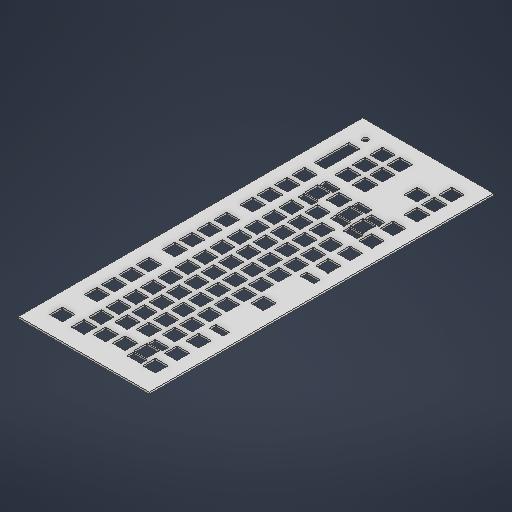
# Autodesk Inventor part: Keyboard-top
Saved by Autodesk Inventor 2026.1 (Build 301233000, 233)
## iProperties
Created: 2025-12-15
Part Number: Keyboard-top
Material: Generic
Document SubType Name: Modeling
Designer: chest
Density: 1 g/cm^3
Appearance: Default
Author: chest
Autodesk Inventor part; units mm, degrees
(part 1 of 5)
ref_plane "YZ Plane" through (0, 0, 0) normal (1, 0, 0) x (0, 1, 0)
ref_plane "XZ Plane" through (0, 0, 0) normal (0, 1, 0) x (-1, 0, 0)
ref_plane "XY Plane" through (0, 0, 0) normal (0, 0, 1) x (1, 0, 0)
sketch "Block1" plane through (0, 0, 0) normal (0, 0, 1) x (1, 0, 0)
  line L0 (31.1, 3.025) -> (31.1, 16.025)
  line L1 (45.1, 3.025) -> (45.1, 16.025)
  line L2 (31.6, 2.525) -> (44.6, 2.525)
  line L3 (31.6, 16.525) -> (44.6, 16.525)
  arc A0 (31.1, 3.025) -> (31.6, 2.525) centre (31.6, 3.025) ccw
  arc A1 (31.6, 16.525) -> (31.1, 16.025) centre (31.6, 16.025) ccw
  arc A2 (44.6, 2.525) -> (45.1, 3.025) centre (44.6, 3.025) ccw
  arc A3 (45.1, 16.025) -> (44.6, 16.525) centre (44.6, 16.025) ccw
  line L4 (31.1, 22.075) -> (31.1, 35.075)
  line L5 (45.1, 22.075) -> (45.1, 35.075)
  line L6 (31.6, 21.575) -> (44.6, 21.575)
  line L7 (31.6, 35.575) -> (44.6, 35.575)
  arc A4 (31.1, 22.075) -> (31.6, 21.575) centre (31.6, 22.075) ccw
  arc A5 (31.6, 35.575) -> (31.1, 35.075) centre (31.6, 35.075) ccw
  arc A6 (44.6, 21.575) -> (45.1, 22.075) centre (44.6, 22.075) ccw
  arc A7 (45.1, 35.075) -> (44.6, 35.575) centre (44.6, 35.075) ccw
  line L8 (31.1, 41.125) -> (31.1, 54.125)
  line L9 (45.1, 41.125) -> (45.1, 54.125)
  line L10 (31.6, 40.625) -> (44.6, 40.625)
  line L11 (31.6, 54.625) -> (44.6, 54.625)
  arc A8 (31.1, 41.125) -> (31.6, 40.625) centre (31.6, 41.125) ccw
  arc A9 (31.6, 54.625) -> (31.1, 54.125) centre (31.6, 54.125) ccw
  arc A10 (44.6, 40.625) -> (45.1, 41.125) centre (44.6, 41.125) ccw
  arc A11 (45.1, 54.125) -> (44.6, 54.625) centre (44.6, 54.125) ccw
  line L12 (31.1, 60.175) -> (31.1, 73.175)
  line L13 (45.1, 60.175) -> (45.1, 73.175)
  line L14 (31.6, 59.675) -> (44.6, 59.675)
  line L15 (31.6, 73.675) -> (44.6, 73.675)
  arc A12 (31.1, 60.175) -> (31.6, 59.675) centre (31.6, 60.175) ccw
  arc A13 (31.6, 73.675) -> (31.1, 73.175) centre (31.6, 73.175) ccw
  arc A14 (44.6, 59.675) -> (45.1, 60.175) centre (44.6, 60.175) ccw
  arc A15 (45.1, 73.175) -> (44.6, 73.675) centre (44.6, 73.175) ccw
  line L16 (31.1, 79.225) -> (31.1, 92.225)
  line L17 (45.1, 79.225) -> (45.1, 92.225)
  line L18 (31.6, 78.725) -> (44.6, 78.725)
  line L19 (31.6, 92.725) -> (44.6, 92.725)
  arc A16 (31.1, 79.225) -> (31.6, 78.725) centre (31.6, 79.225) ccw
  arc A17 (31.6, 92.725) -> (31.1, 92.225) centre (31.6, 92.225) ccw
  arc A18 (44.6, 78.725) -> (45.1, 79.225) centre (44.6, 79.225) ccw
  arc A19 (45.1, 92.225) -> (44.6, 92.725) centre (44.6, 92.225) ccw
  line L20 (31.1, 98.275) -> (31.1, 111.275)
  line L21 (45.1, 98.275) -> (45.1, 111.275)
  line L22 (31.6, 97.775) -> (44.6, 97.775)
  line L23 (31.6, 111.775) -> (44.6, 111.775)
  arc A20 (31.1, 98.275) -> (31.6, 97.775) centre (31.6, 98.275) ccw
  arc A21 (31.6, 111.775) -> (31.1, 111.275) centre (31.6, 111.275) ccw
  arc A22 (44.6, 97.775) -> (45.1, 98.275) centre (44.6, 98.275) ccw
  arc A23 (45.1, 111.275) -> (44.6, 111.775) centre (44.6, 111.275) ccw
  line L24 (31.1, 117.325) -> (31.1, 130.325)
  line L25 (45.1, 117.325) -> (45.1, 130.325)
  line L26 (31.6, 116.825) -> (44.6, 116.825)
  line L27 (31.6, 130.825) -> (44.6, 130.825)
  arc A24 (31.1, 117.325) -> (31.6, 116.825) centre (31.6, 117.325) ccw
  arc A25 (31.6, 130.825) -> (31.1, 130.325) centre (31.6, 130.325) ccw
  arc A26 (44.6, 116.825) -> (45.1, 117.325) centre (44.6, 117.325) ccw
  arc A27 (45.1, 130.325) -> (44.6, 130.825) centre (44.6, 130.325) ccw
  line L28 (31.1, 136.375) -> (31.1, 149.375)
  line L29 (45.1, 136.375) -> (45.1, 149.375)
  line L30 (31.6, 135.875) -> (44.6, 135.875)
  line L31 (31.6, 149.875) -> (44.6, 149.875)
  arc A28 (31.1, 136.375) -> (31.6, 135.875) centre (31.6, 136.375) ccw
  arc A29 (31.6, 149.875) -> (31.1, 149.375) centre (31.6, 149.375) ccw
  arc A30 (44.6, 135.875) -> (45.1, 136.375) centre (44.6, 136.375) ccw
  arc A31 (45.1, 149.375) -> (44.6, 149.875) centre (44.6, 149.375) ccw
  line L32 (31.1, 155.425) -> (31.1, 168.425)
  line L33 (45.1, 155.425) -> (45.1, 168.425)
  line L34 (31.6, 154.925) -> (44.6, 154.925)
  line L35 (31.6, 168.925) -> (44.6, 168.925)
  arc A32 (31.1, 155.425) -> (31.6, 154.925) centre (31.6, 155.425) ccw
  arc A33 (31.6, 168.925) -> (31.1, 168.425) centre (31.6, 168.425) ccw
  arc A34 (44.6, 154.925) -> (45.1, 155.425) centre (44.6, 155.425) ccw
  arc A35 (45.1, 168.425) -> (44.6, 168.925) centre (44.6, 168.425) ccw
  line L36 (31.1, 174.475) -> (31.1, 187.475)
  line L37 (45.1, 174.475) -> (45.1, 187.475)
  line L38 (31.6, 173.975) -> (44.6, 173.975)
  line L39 (31.6, 187.975) -> (44.6, 187.975)
  arc A36 (31.1, 174.475) -> (31.6, 173.975) centre (31.6, 174.475) ccw
  arc A37 (31.6, 187.975) -> (31.1, 187.475) centre (31.6, 187.475) ccw
  arc A38 (44.6, 173.975) -> (45.1, 174.475) centre (44.6, 174.475) ccw
  arc A39 (45.1, 187.475) -> (44.6, 187.975) centre (44.6, 187.475) ccw
  line L40 (31.1, 193.525) -> (31.1, 206.525)
  line L41 (45.1, 193.525) -> (45.1, 206.525)
  line L42 (31.6, 193.025) -> (44.6, 193.025)
  line L43 (31.6, 207.025) -> (44.6, 207.025)
  arc A40 (31.1, 193.525) -> (31.6, 193.025) centre (31.6, 193.525) ccw
  arc A41 (31.6, 207.025) -> (31.1, 206.525) centre (31.6, 206.525) ccw
  arc A42 (44.6, 193.025) -> (45.1, 193.525) centre (44.6, 193.525) ccw
  arc A43 (45.1, 206.525) -> (44.6, 207.025) centre (44.6, 206.525) ccw
  line L44 (31.1, 212.575) -> (31.1, 225.575)
  line L45 (45.1, 212.575) -> (45.1, 225.575)
  line L46 (31.6, 212.075) -> (44.6, 212.075)
  line L47 (31.6, 226.075) -> (44.6, 226.075)
  arc A44 (31.1, 212.575) -> (31.6, 212.075) centre (31.6, 212.575) ccw
  arc A45 (31.6, 226.075) -> (31.1, 225.575) centre (31.6, 225.575) ccw
  arc A46 (44.6, 212.075) -> (45.1, 212.575) centre (44.6, 212.575) ccw
  arc A47 (45.1, 225.575) -> (44.6, 226.075) centre (44.6, 225.575) ccw
  line L48 (31.1, 231.625) -> (31.1, 244.625)
  line L49 (45.1, 231.625) -> (45.1, 244.625)
  line L50 (31.6, 231.125) -> (44.6, 231.125)
  line L51 (31.6, 245.125) -> (44.6, 245.125)
  arc A48 (31.1, 231.625) -> (31.6, 231.125) centre (31.6, 231.625) ccw
  arc A49 (31.6, 245.125) -> (31.1, 244.625) centre (31.6, 244.625) ccw
  arc A50 (44.6, 231.125) -> (45.1, 231.625) centre (44.6, 231.625) ccw
  arc A51 (45.1, 244.625) -> (44.6, 245.125) centre (44.6, 244.625) ccw
  line L52 (31.1, 260.2) -> (31.1, 273.2)
  line L53 (45.1, 260.2) -> (45.1, 273.2)
  line L54 (31.6, 259.7) -> (44.6, 259.7)
  line L55 (31.6, 273.7) -> (44.6, 273.7)
  arc A52 (31.1, 260.2) -> (31.6, 259.7) centre (31.6, 260.2) ccw
  arc A53 (31.6, 273.7) -> (31.1, 273.2) centre (31.6, 273.2) ccw
  arc A54 (44.6, 259.7) -> (45.1, 260.2) centre (44.6, 260.2) ccw
  arc A55 (45.1, 273.2) -> (44.6, 273.7) centre (44.6, 273.2) ccw
  line L56 (32.1, 251.762) -> (32.1, 257.762)
  line L57 (47.1, 251.762) -> (47.1, 257.762)
  line L58 (32.6, 251.262) -> (46.6, 251.262)
  line L59 (32.6, 258.262) -> (46.6, 258.262)
  arc A56 (32.1, 251.762) -> (32.6, 251.262) centre (32.6, 251.762) ccw
  arc A57 (32.6, 258.262) -> (32.1, 257.762) centre (32.6, 257.762) ccw
  arc A58 (46.6, 251.262) -> (47.1, 251.762) centre (46.6, 251.762) ccw
  arc A59 (47.1, 257.762) -> (46.6, 258.262) centre (46.6, 257.762) ccw
  line L60 (32.1, 275.638) -> (32.1, 281.638)
  line L61 (47.1, 275.638) -> (47.1, 281.638)
  line L62 (32.6, 275.138) -> (46.6, 275.138)
  line L63 (32.6, 282.138) -> (46.6, 282.138)
  arc A60 (32.1, 275.638) -> (32.6, 275.138) centre (32.6, 275.638) ccw
  arc A61 (32.6, 282.138) -> (32.1, 281.638) centre (32.6, 281.638) ccw
  arc A62 (46.6, 275.138) -> (47.1, 275.638) centre (46.6, 275.638) ccw
  arc A63 (47.1, 281.638) -> (46.6, 282.138) centre (46.6, 281.638) ccw
  line L64 (31.1, 293.5375) -> (31.1, 306.5375)
  line L65 (45.1, 293.5375) -> (45.1, 306.5375)
  line L66 (31.6, 293.0375) -> (44.6, 293.0375)
  line L67 (31.6, 307.0375) -> (44.6, 307.0375)
  arc A64 (31.1, 293.5375) -> (31.6, 293.0375) centre (31.6, 293.5375) ccw
  arc A65 (31.6, 307.0375) -> (31.1, 306.5375) centre (31.6, 306.5375) ccw
  arc A66 (44.6, 293.0375) -> (45.1, 293.5375) centre (44.6, 293.5375) ccw
  arc A67 (45.1, 306.5375) -> (44.6, 307.0375) centre (44.6, 306.5375) ccw
  line L68 (31.1, 312.5875) -> (31.1, 325.5875)
  line L69 (45.1, 312.5875) -> (45.1, 325.5875)
  line L70 (31.6, 312.0875) -> (44.6, 312.0875)
  line L71 (31.6, 326.0875) -> (44.6, 326.0875)
  arc A68 (31.1, 312.5875) -> (31.6, 312.0875) centre (31.6, 312.5875) ccw
  arc A69 (31.6, 326.0875) -> (31.1, 325.5875) centre (31.6, 325.5875) ccw
  arc A70 (44.6, 312.0875) -> (45.1, 312.5875) centre (44.6, 312.5875) ccw
  arc A71 (45.1, 325.5875) -> (44.6, 326.0875) centre (44.6, 325.5875) ccw
  line L72 (31.1, 331.6375) -> (31.1, 344.6375)
  line L73 (45.1, 331.6375) -> (45.1, 344.6375)
  line L74 (31.6, 331.1375) -> (44.6, 331.1375)
  line L75 (31.6, 345.1375) -> (44.6, 345.1375)
  arc A72 (31.1, 331.6375) -> (31.6, 331.1375) centre (31.6, 331.6375) ccw
  arc A73 (31.6, 345.1375) -> (31.1, 344.6375) centre (31.6, 344.6375) ccw
  arc A74 (44.6, 331.1375) -> (45.1, 331.6375) centre (44.6, 331.6375) ccw
  arc A75 (45.1, 344.6375) -> (44.6, 345.1375) centre (44.6, 344.6375) ccw
  line L76 (50.15, 7.7875) -> (50.15, 20.7875)
  line L77 (64.15, 7.7875) -> (64.15, 20.7875)
  line L78 (50.65, 7.2875) -> (63.65, 7.2875)
  line L79 (50.65, 21.2875) -> (63.65, 21.2875)
  arc A76 (50.15, 7.7875) -> (50.65, 7.2875) centre (50.65, 7.7875) ccw
  arc A77 (50.65, 21.2875) -> (50.15, 20.7875) centre (50.65, 20.7875) ccw
  arc A78 (63.65, 7.2875) -> (64.15, 7.7875) centre (63.65, 7.7875) ccw
  arc A79 (64.15, 20.7875) -> (63.65, 21.2875) centre (63.65, 20.7875) ccw
  line L80 (50.15, 31.6) -> (50.15, 44.6)
  line L81 (64.15, 31.6) -> (64.15, 44.6)
  line L82 (50.65, 31.1) -> (63.65, 31.1)
  line L83 (50.65, 45.1) -> (63.65, 45.1)
  arc A80 (50.15, 31.6) -> (50.65, 31.1) centre (50.65, 31.6) ccw
  arc A81 (50.65, 45.1) -> (50.15, 44.6) centre (50.65, 44.6) ccw
  arc A82 (63.65, 31.1) -> (64.15, 31.6) centre (63.65, 31.6) ccw
  arc A83 (64.15, 44.6) -> (63.65, 45.1) centre (63.65, 44.6) ccw
  line L84 (50.15, 50.65) -> (50.15, 63.65)
  line L85 (64.15, 50.65) -> (64.15, 63.65)
  line L86 (50.65, 50.15) -> (63.65, 50.15)
  line L87 (50.65, 64.15) -> (63.65, 64.15)
  arc A84 (50.15, 50.65) -> (50.65, 50.15) centre (50.65, 50.65) ccw
  arc A85 (50.65, 64.15) -> (50.15, 63.65) centre (50.65, 63.65) ccw
  arc A86 (63.65, 50.15) -> (64.15, 50.65) centre (63.65, 50.65) ccw
  arc A87 (64.15, 63.65) -> (63.65, 64.15) centre (63.65, 63.65) ccw
  line L88 (50.15, 69.7) -> (50.15, 82.7)
  line L89 (64.15, 69.7) -> (64.15, 82.7)
  line L90 (50.65, 69.2) -> (63.65, 69.2)
  line L91 (50.65, 83.2) -> (63.65, 83.2)
  arc A88 (50.15, 69.7) -> (50.65, 69.2) centre (50.65, 69.7) ccw
  arc A89 (50.65, 83.2) -> (50.15, 82.7) centre (50.65, 82.7) ccw
  arc A90 (63.65, 69.2) -> (64.15, 69.7) centre (63.65, 69.7) ccw
  arc A91 (64.15, 82.7) -> (63.65, 83.2) centre (63.65, 82.7) ccw
  line L92 (50.15, 88.75) -> (50.15, 101.75)
  line L93 (64.15, 88.75) -> (64.15, 101.75)
  line L94 (50.65, 88.25) -> (63.65, 88.25)
  line L95 (50.65, 102.25) -> (63.65, 102.25)
  arc A92 (50.15, 88.75) -> (50.65, 88.25) centre (50.65, 88.75) ccw
  arc A93 (50.65, 102.25) -> (50.15, 101.75) centre (50.65, 101.75) ccw
  arc A94 (63.65, 88.25) -> (64.15, 88.75) centre (63.65, 88.75) ccw
  arc A95 (64.15, 101.75) -> (63.65, 102.25) centre (63.65, 101.75) ccw
  line L96 (50.15, 107.8) -> (50.15, 120.8)
  line L97 (64.15, 107.8) -> (64.15, 120.8)
  line L98 (50.65, 107.3) -> (63.65, 107.3)
  line L99 (50.65, 121.3) -> (63.65, 121.3)
  arc A96 (50.15, 107.8) -> (50.65, 107.3) centre (50.65, 107.8) ccw
  arc A97 (50.65, 121.3) -> (50.15, 120.8) centre (50.65, 120.8) ccw
  arc A98 (63.65, 107.3) -> (64.15, 107.8) centre (63.65, 107.8) ccw
  arc A99 (64.15, 120.8) -> (63.65, 121.3) centre (63.65, 120.8) ccw
  line L100 (50.15, 126.85) -> (50.15, 139.85)
  line L101 (64.15, 126.85) -> (64.15, 139.85)
  line L102 (50.65, 126.35) -> (63.65, 126.35)
  line L103 (50.65, 140.35) -> (63.65, 140.35)
  arc A100 (50.15, 126.85) -> (50.65, 126.35) centre (50.65, 126.85) ccw
  arc A101 (50.65, 140.35) -> (50.15, 139.85) centre (50.65, 139.85) ccw
  arc A102 (63.65, 126.35) -> (64.15, 126.85) centre (63.65, 126.85) ccw
  arc A103 (64.15, 139.85) -> (63.65, 140.35) centre (63.65, 139.85) ccw
  line L104 (50.15, 145.9) -> (50.15, 158.9)
  line L105 (64.15, 145.9) -> (64.15, 158.9)
  line L106 (50.65, 145.4) -> (63.65, 145.4)
  line L107 (50.65, 159.4) -> (63.65, 159.4)
  arc A104 (50.15, 145.9) -> (50.65, 145.4) centre (50.65, 145.9) ccw
  arc A105 (50.65, 159.4) -> (50.15, 158.9) centre (50.65, 158.9) ccw
  arc A106 (63.65, 145.4) -> (64.15, 145.9) centre (63.65, 145.9) ccw
  arc A107 (64.15, 158.9) -> (63.65, 159.4) centre (63.65, 158.9) ccw
  line L108 (50.15, 164.95) -> (50.15, 177.95)
  line L109 (64.15, 164.95) -> (64.15, 177.95)
  line L110 (50.65, 164.45) -> (63.65, 164.45)
  line L111 (50.65, 178.45) -> (63.65, 178.45)
  arc A108 (50.15, 164.95) -> (50.65, 164.45) centre (50.65, 164.95) ccw
  arc A109 (50.65, 178.45) -> (50.15, 177.95) centre (50.65, 177.95) ccw
  arc A110 (63.65, 164.45) -> (64.15, 164.95) centre (63.65, 164.95) ccw
  arc A111 (64.15, 177.95) -> (63.65, 178.45) centre (63.65, 177.95) ccw
  line L112 (50.15, 184) -> (50.15, 197)
  line L113 (64.15, 184) -> (64.15, 197)
  line L114 (50.65, 183.5) -> (63.65, 183.5)
  line L115 (50.65, 197.5) -> (63.65, 197.5)
  arc A112 (50.15, 184) -> (50.65, 183.5) centre (50.65, 184) ccw
  arc A113 (50.65, 197.5) -> (50.15, 197) centre (50.65, 197) ccw
  arc A114 (63.65, 183.5) -> (64.15, 184) centre (63.65, 184) ccw
  arc A115 (64.15, 197) -> (63.65, 197.5) centre (63.65, 197) ccw
  line L116 (50.15, 203.05) -> (50.15, 216.05)
  line L117 (64.15, 203.05) -> (64.15, 216.05)
  line L118 (50.65, 202.55) -> (63.65, 202.55)
  line L119 (50.65, 216.55) -> (63.65, 216.55)
  arc A116 (50.15, 203.05) -> (50.65, 202.55) centre (50.65, 203.05) ccw
  arc A117 (50.65, 216.55) -> (50.15, 216.05) centre (50.65, 216.05) ccw
  arc A118 (63.65, 202.55) -> (64.15, 203.05) centre (63.65, 203.05) ccw
  arc A119 (64.15, 216.05) -> (63.65, 216.55) centre (63.65, 216.05) ccw
  line L120 (50.15, 222.1) -> (50.15, 235.1)
  line L121 (64.15, 222.1) -> (64.15, 235.1)
  line L122 (50.65, 221.6) -> (63.65, 221.6)
  line L123 (50.65, 235.6) -> (63.65, 235.6)
  arc A120 (50.15, 222.1) -> (50.65, 221.6) centre (50.65, 222.1) ccw
  arc A121 (50.65, 235.6) -> (50.15, 235.1) centre (50.65, 235.1) ccw
  arc A122 (63.65, 221.6) -> (64.15, 222.1) centre (63.65, 222.1) ccw
  arc A123 (64.15, 235.1) -> (63.65, 235.6) centre (63.65, 235.1) ccw
  line L124 (50.15, 241.15) -> (50.15, 254.15)
  line L125 (64.15, 241.15) -> (64.15, 254.15)
  line L126 (50.65, 240.65) -> (63.65, 240.65)
  line L127 (50.65, 254.65) -> (63.65, 254.65)
  arc A124 (50.15, 241.15) -> (50.65, 240.65) centre (50.65, 241.15) ccw
  arc A125 (50.65, 254.65) -> (50.15, 254.15) centre (50.65, 254.15) ccw
  arc A126 (63.65, 240.65) -> (64.15, 241.15) centre (63.65, 241.15) ccw
  arc A127 (64.15, 254.15) -> (63.65, 254.65) centre (63.65, 254.15) ccw
  line L128 (50.15, 264.9625) -> (50.15, 277.9625)
  line L129 (64.15, 264.9625) -> (64.15, 277.9625)
  line L130 (50.65, 264.4625) -> (63.65, 264.4625)
  line L131 (50.65, 278.4625) -> (63.65, 278.4625)
  arc A128 (50.15, 264.9625) -> (50.65, 264.4625) centre (50.65, 264.9625) ccw
  arc A129 (50.65, 278.4625) -> (50.15, 277.9625) centre (50.65, 277.9625) ccw
  arc A130 (63.65, 264.4625) -> (64.15, 264.9625) centre (63.65, 264.9625) ccw
  arc A131 (64.15, 277.9625) -> (63.65, 278.4625) centre (63.65, 277.9625) ccw
  line L132 (50.15, 293.5375) -> (50.15, 306.5375)
  line L133 (64.15, 293.5375) -> (64.15, 306.5375)
  line L134 (50.65, 293.0375) -> (63.65, 293.0375)
  line L135 (50.65, 307.0375) -> (63.65, 307.0375)
  arc A132 (50.15, 293.5375) -> (50.65, 293.0375) centre (50.65, 293.5375) ccw
  arc A133 (50.65, 307.0375) -> (50.15, 306.5375) centre (50.65, 306.5375) ccw
  arc A134 (63.65, 293.0375) -> (64.15, 293.5375) centre (63.65, 293.5375) ccw
  arc A135 (64.15, 306.5375) -> (63.65, 307.0375) centre (63.65, 306.5375) ccw
  line L136 (50.15, 312.5875) -> (50.15, 325.5875)
  line L137 (64.15, 312.5875) -> (64.15, 325.5875)
  line L138 (50.65, 312.0875) -> (63.65, 312.0875)
  line L139 (50.65, 326.0875) -> (63.65, 326.0875)
  arc A136 (50.15, 312.5875) -> (50.65, 312.0875) centre (50.65, 312.5875) ccw
  arc A137 (50.65, 326.0875) -> (50.15, 325.5875) centre (50.65, 325.5875) ccw
  arc A138 (63.65, 312.0875) -> (64.15, 312.5875) centre (63.65, 312.5875) ccw
  arc A139 (64.15, 325.5875) -> (63.65, 326.0875) centre (63.65, 325.5875) ccw
  line L140 (50.15, 331.6375) -> (50.15, 344.6375)
  line L141 (64.15, 331.6375) -> (64.15, 344.6375)
  line L142 (50.65, 331.1375) -> (63.65, 331.1375)
  line L143 (50.65, 345.1375) -> (63.65, 345.1375)
  arc A140 (50.15, 331.6375) -> (50.65, 331.1375) centre (50.65, 331.6375) ccw
  arc A141 (50.65, 345.1375) -> (50.15, 344.6375) centre (50.65, 344.6375) ccw
  arc A142 (63.65, 331.1375) -> (64.15, 331.6375) centre (63.65, 331.6375) ccw
  arc A143 (64.15, 344.6375) -> (63.65, 345.1375) centre (63.65, 344.6375) ccw
  line L144 (69.2, 10.1688) -> (69.2, 23.1688)
  line L145 (83.2, 10.1687) -> (83.2, 23.1688)
  line L146 (69.7, 9.6687) -> (82.7, 9.6688)
  line L147 (69.7, 23.6687) -> (82.7, 23.6688)
  arc A144 (69.2, 10.1688) -> (69.7, 9.6687) centre (69.7, 10.1687) ccw
  arc A145 (69.7, 23.6687) -> (69.2, 23.1688) centre (69.7, 23.1687) ccw
  arc A146 (82.7, 9.6687) -> (83.2, 10.1687) centre (82.7, 10.1687) ccw
  arc A147 (83.2, 23.1687) -> (82.7, 23.6688) centre (82.7, 23.1687) ccw
  line L148 (69.2, 36.3625) -> (69.2, 49.3625)
  line L149 (83.2, 36.3625) -> (83.2, 49.3625)
  line L150 (69.7, 35.8625) -> (82.7, 35.8625)
  line L151 (69.7, 49.8625) -> (82.7, 49.8625)
  arc A148 (69.2, 36.3625) -> (69.7, 35.8625) centre (69.7, 36.3625) ccw
  arc A149 (69.7, 49.8625) -> (69.2, 49.3625) centre (69.7, 49.3625) ccw
  arc A150 (82.7, 35.8625) -> (83.2, 36.3625) centre (82.7, 36.3625) ccw
  arc A151 (83.2, 49.3625) -> (82.7, 49.8625) centre (82.7, 49.3625) ccw
  line L152 (69.2, 55.4125) -> (69.2, 68.4125)
  line L153 (83.2, 55.4125) -> (83.2, 68.4125)
  line L154 (69.7, 54.9125) -> (82.7, 54.9125)
  line L155 (69.7, 68.9125) -> (82.7, 68.9125)
  arc A152 (69.2, 55.4125) -> (69.7, 54.9125) centre (69.7, 55.4125) ccw
  arc A153 (69.7, 68.9125) -> (69.2, 68.4125) centre (69.7, 68.4125) ccw
  arc A154 (82.7, 54.9125) -> (83.2, 55.4125) centre (82.7, 55.4125) ccw
  arc A155 (83.2, 68.4125) -> (82.7, 68.9125) centre (82.7, 68.4125) ccw
  line L156 (69.2, 74.4625) -> (69.2, 87.4625)
  line L157 (83.2, 74.4625) -> (83.2, 87.4625)
  line L158 (69.7, 73.9625) -> (82.7, 73.9625)
  line L159 (69.7, 87.9625) -> (82.7, 87.9625)
  arc A156 (69.2, 74.4625) -> (69.7, 73.9625) centre (69.7, 74.4625) ccw
  arc A157 (69.7, 87.9625) -> (69.2, 87.4625) centre (69.7, 87.4625) ccw
  arc A158 (82.7, 73.9625) -> (83.2, 74.4625) centre (82.7, 74.4625) ccw
  arc A159 (83.2, 87.4625) -> (82.7, 87.9625) centre (82.7, 87.4625) ccw
  line L160 (69.2, 93.5125) -> (69.2, 106.5125)
  line L161 (83.2, 93.5125) -> (83.2, 106.5125)
  line L162 (69.7, 93.0125) -> (82.7, 93.0125)
  line L163 (69.7, 107.0125) -> (82.7, 107.0125)
  arc A160 (69.2, 93.5125) -> (69.7, 93.0125) centre (69.7, 93.5125) ccw
  arc A161 (69.7, 107.0125) -> (69.2, 106.5125) centre (69.7, 106.5125) ccw
  arc A162 (82.7, 93.0125) -> (83.2, 93.5125) centre (82.7, 93.5125) ccw
  arc A163 (83.2, 106.5125) -> (82.7, 107.0125) centre (82.7, 106.5125) ccw
  line L164 (69.2, 112.5625) -> (69.2, 125.5625)
  line L165 (83.2, 112.5625) -> (83.2, 125.5625)
  line L166 (69.7, 112.0625) -> (82.7, 112.0625)
  line L167 (69.7, 126.0625) -> (82.7, 126.0625)
  arc A164 (69.2, 112.5625) -> (69.7, 112.0625) centre (69.7, 112.5625) ccw
  arc A165 (69.7, 126.0625) -> (69.2, 125.5625) centre (69.7, 125.5625) ccw
  arc A166 (82.7, 112.0625) -> (83.2, 112.5625) centre (82.7, 112.5625) ccw
  arc A167 (83.2, 125.5625) -> (82.7, 126.0625) centre (82.7, 125.5625) ccw
  line L168 (69.2, 131.6125) -> (69.2, 144.6125)
  line L169 (83.2, 131.6125) -> (83.2, 144.6125)
  line L170 (69.7, 131.1125) -> (82.7, 131.1125)
  line L171 (69.7, 145.1125) -> (82.7, 145.1125)
  arc A168 (69.2, 131.6125) -> (69.7, 131.1125) centre (69.7, 131.6125) ccw
  arc A169 (69.7, 145.1125) -> (69.2, 144.6125) centre (69.7, 144.6125) ccw
  arc A170 (82.7, 131.1125) -> (83.2, 131.6125) centre (82.7, 131.6125) ccw
  arc A171 (83.2, 144.6125) -> (82.7, 145.1125) centre (82.7, 144.6125) ccw
  line L172 (69.2, 150.6625) -> (69.2, 163.6625)
  line L173 (83.2, 150.6625) -> (83.2, 163.6625)
  line L174 (69.7, 150.1625) -> (82.7, 150.1625)
  line L175 (69.7, 164.1625) -> (82.7, 164.1625)
  arc A172 (69.2, 150.6625) -> (69.7, 150.1625) centre (69.7, 150.6625) ccw
  arc A173 (69.7, 164.1625) -> (69.2, 163.6625) centre (69.7, 163.6625) ccw
  arc A174 (82.7, 150.1625) -> (83.2, 150.6625) centre (82.7, 150.6625) ccw
  arc A175 (83.2, 163.6625) -> (82.7, 164.1625) centre (82.7, 163.6625) ccw
  line L176 (69.2, 169.7125) -> (69.2, 182.7125)
  line L177 (83.2, 169.7125) -> (83.2, 182.7125)
  line L178 (69.7, 169.2125) -> (82.7, 169.2125)
  line L179 (69.7, 183.2125) -> (82.7, 183.2125)
  arc A176 (69.2, 169.7125) -> (69.7, 169.2125) centre (69.7, 169.7125) ccw
  arc A177 (69.7, 183.2125) -> (69.2, 182.7125) centre (69.7, 182.7125) ccw
  arc A178 (82.7, 169.2125) -> (83.2, 169.7125) centre (82.7, 169.7125) ccw
  arc A179 (83.2, 182.7125) -> (82.7, 183.2125) centre (82.7, 182.7125) ccw
  line L180 (69.2, 188.7625) -> (69.2, 201.7625)
  line L181 (83.2, 188.7625) -> (83.2, 201.7625)
  line L182 (69.7, 188.2625) -> (82.7, 188.2625)
  line L183 (69.7, 202.2625) -> (82.7, 202.2625)
  arc A180 (69.2, 188.7625) -> (69.7, 188.2625) centre (69.7, 188.7625) ccw
  arc A181 (69.7, 202.2625) -> (69.2, 201.7625) centre (69.7, 201.7625) ccw
  arc A182 (82.7, 188.2625) -> (83.2, 188.7625) centre (82.7, 188.7625) ccw
  arc A183 (83.2, 201.7625) -> (82.7, 202.2625) centre (82.7, 201.7625) ccw
  line L184 (69.2, 207.8125) -> (69.2, 220.8125)
  line L185 (83.2, 207.8125) -> (83.2, 220.8125)
  line L186 (69.7, 207.3125) -> (82.7, 207.3125)
  line L187 (69.7, 221.3125) -> (82.7, 221.3125)
  arc A184 (69.2, 207.8125) -> (69.7, 207.3125) centre (69.7, 207.8125) ccw
  arc A185 (69.7, 221.3125) -> (69.2, 220.8125) centre (69.7, 220.8125) ccw
  arc A186 (82.7, 207.3125) -> (83.2, 207.8125) centre (82.7, 207.8125) ccw
  arc A187 (83.2, 220.8125) -> (82.7, 221.3125) centre (82.7, 220.8125) ccw
  line L188 (69.2, 226.8625) -> (69.2, 239.8625)
  line L189 (83.2, 226.8625) -> (83.2, 239.8625)
  line L190 (69.7, 226.3625) -> (82.7, 226.3625)
  line L191 (69.7, 240.3625) -> (82.7, 240.3625)
  arc A188 (69.2, 226.8625) -> (69.7, 226.3625) centre (69.7, 226.8625) ccw
  arc A189 (69.7, 240.3625) -> (69.2, 239.8625) centre (69.7, 239.8625) ccw
  arc A190 (82.7, 226.3625) -> (83.2, 226.8625) centre (82.7, 226.8625) ccw
  arc A191 (83.2, 239.8625) -> (82.7, 240.3625) centre (82.7, 239.8625) ccw
  line L192 (69.2, 257.8188) -> (69.2, 270.8188)
  line L193 (83.2, 257.8188) -> (83.2, 270.8188)
  line L194 (69.7, 257.3188) -> (82.7, 257.3188)
  line L195 (69.7, 271.3188) -> (82.7, 271.3188)
  arc A192 (69.2, 257.8188) -> (69.7, 257.3188) centre (69.7, 257.8188) ccw
  arc A193 (69.7, 271.3188) -> (69.2, 270.8188) centre (69.7, 270.8188) ccw
  arc A194 (82.7, 257.3188) -> (83.2, 257.8188) centre (82.7, 257.8188) ccw
  arc A195 (83.2, 270.8188) -> (82.7, 271.3188) centre (82.7, 270.8188) ccw
  line L196 (70.2, 249.3808) -> (70.2, 255.3808)
  line L197 (85.2, 249.3808) -> (85.2, 255.3808)
  line L198 (70.7, 248.8808) -> (84.7, 248.8808)
  line L199 (70.7, 255.8808) -> (84.7, 255.8808)
  arc A196 (70.2, 249.3808) -> (70.7, 248.8808) centre (70.7, 249.3808) ccw
  arc A197 (70.7, 255.8808) -> (70.2, 255.3808) centre (70.7, 255.3808) ccw
  arc A198 (84.7, 248.8808) -> (85.2, 249.3808) centre (84.7, 249.3808) ccw
  arc A199 (85.2, 255.3808) -> (84.7, 255.8808) centre (84.7, 255.3808) ccw
  line L200 (70.2, 273.2568) -> (70.2, 279.2568)
  line L201 (85.2, 273.2568) -> (85.2, 279.2568)
  line L202 (70.7, 272.7568) -> (84.7, 272.7568)
  line L203 (70.7, 279.7568) -> (84.7, 279.7568)
  arc A200 (70.2, 273.2568) -> (70.7, 272.7568) centre (70.7, 273.2568) ccw
  arc A201 (70.7, 279.7568) -> (70.2, 279.2568) centre (70.7, 279.2568) ccw
  arc A202 (84.7, 272.7568) -> (85.2, 273.2568) centre (84.7, 273.2568) ccw
  arc A203 (85.2, 279.2568) -> (84.7, 279.7568) centre (84.7, 279.2568) ccw
  line L204 (88.25, 14.9313) -> (88.25, 27.9313)
  line L205 (102.25, 14.9313) -> (102.25, 27.9312)
  line L206 (88.75, 14.4312) -> (101.75, 14.4313)
  line L207 (88.75, 28.4313) -> (101.75, 28.4313)
  arc A204 (88.25, 14.9313) -> (88.75, 14.4312) centre (88.75, 14.9313) ccw
  arc A205 (88.75, 28.4313) -> (88.25, 27.9313) centre (88.75, 27.9312) ccw
  arc A206 (101.75, 14.4313) -> (102.25, 14.9312) centre (101.75, 14.9313) ccw
  arc A207 (102.25, 27.9312) -> (101.75, 28.4312) centre (101.75, 27.9312) ccw
  line L208 (89.25, 6.4933) -> (89.25, 12.4933)
  line L209 (104.25, 6.4932) -> (104.25, 12.4932)
  line L210 (89.75, 5.9933) -> (103.75, 5.9932)
  line L211 (89.75, 12.9933) -> (103.75, 12.9932)
  arc A208 (89.25, 6.4933) -> (89.75, 5.9933) centre (89.75, 6.4932) ccw
  arc A209 (89.75, 12.9933) -> (89.25, 12.4933) centre (89.75, 12.4933) ccw
  arc A210 (103.75, 5.9932) -> (104.25, 6.4932) centre (103.75, 6.4933) ccw
  arc A211 (104.25, 12.4932) -> (103.75, 12.9932) centre (103.75, 12.4932) ccw
  line L212 (89.25, 30.3693) -> (89.25, 36.3693)
  line L213 (104.25, 30.3693) -> (104.25, 36.3692)
  line L214 (89.75, 29.8692) -> (103.75, 29.8693)
  line L215 (89.75, 36.8693) -> (103.75, 36.8693)
  arc A212 (89.25, 30.3693) -> (89.75, 29.8693) centre (89.75, 30.3693) ccw
  arc A213 (89.75, 36.8693) -> (89.25, 36.3693) centre (89.75, 36.3693) ccw
  arc A214 (103.75, 29.8693) -> (104.25, 30.3693) centre (103.75, 30.3693) ccw
  arc A215 (104.25, 36.3693) -> (103.75, 36.8693) centre (103.75, 36.3693) ccw
  line L216 (88.25, 45.8875) -> (88.25, 58.8875)
  line L217 (102.25, 45.8875) -> (102.25, 58.8875)
  line L218 (88.75, 45.3875) -> (101.75, 45.3875)
  line L219 (88.75, 59.3875) -> (101.75, 59.3875)
  arc A216 (88.25, 45.8875) -> (88.75, 45.3875) centre (88.75, 45.8875) ccw
  arc A217 (88.75, 59.3875) -> (88.25, 58.8875) centre (88.75, 58.8875) ccw
  arc A218 (101.75, 45.3875) -> (102.25, 45.8875) centre (101.75, 45.8875) ccw
  arc A219 (102.25, 58.8875) -> (101.75, 59.3875) centre (101.75, 58.8875) ccw
  line L220 (88.25, 64.9375) -> (88.25, 77.9375)
  line L221 (102.25, 64.9375) -> (102.25, 77.9375)
  line L222 (88.75, 64.4375) -> (101.75, 64.4375)
  line L223 (88.75, 78.4375) -> (101.75, 78.4375)
  arc A220 (88.25, 64.9375) -> (88.75, 64.4375) centre (88.75, 64.9375) ccw
  arc A221 (88.75, 78.4375) -> (88.25, 77.9375) centre (88.75, 77.9375) ccw
  arc A222 (101.75, 64.4375) -> (102.25, 64.9375) centre (101.75, 64.9375) ccw
  arc A223 (102.25, 77.9375) -> (101.75, 78.4375) centre (101.75, 77.9375) ccw
  line L224 (88.25, 83.9875) -> (88.25, 96.9875)
  line L225 (102.25, 83.9875) -> (102.25, 96.9875)
  line L226 (88.75, 83.4875) -> (101.75, 83.4875)
  line L227 (88.75, 97.4875) -> (101.75, 97.4875)
  arc A224 (88.25, 83.9875) -> (88.75, 83.4875) centre (88.75, 83.9875) ccw
  arc A225 (88.75, 97.4875) -> (88.25, 96.9875) centre (88.75, 96.9875) ccw
  arc A226 (101.75, 83.4875) -> (102.25, 83.9875) centre (101.75, 83.9875) ccw
  arc A227 (102.25, 96.9875) -> (101.75, 97.4875) centre (101.75, 96.9875) ccw
  line L228 (88.25, 103.0375) -> (88.25, 116.0375)
  line L229 (102.25, 103.0375) -> (102.25, 116.0375)
  line L230 (88.75, 102.5375) -> (101.75, 102.5375)
  line L231 (88.75, 116.5375) -> (101.75, 116.5375)
  arc A228 (88.25, 103.0375) -> (88.75, 102.5375) centre (88.75, 103.0375) ccw
  arc A229 (88.75, 116.5375) -> (88.25, 116.0375) centre (88.75, 116.0375) ccw
  arc A230 (101.75, 102.5375) -> (102.25, 103.0375) centre (101.75, 103.0375) ccw
  arc A231 (102.25, 116.0375) -> (101.75, 116.5375) centre (101.75, 116.0375) ccw
  line L232 (88.25, 122.0875) -> (88.25, 135.0875)
  line L233 (102.25, 122.0875) -> (102.25, 135.0875)
  line L234 (88.75, 121.5875) -> (101.75, 121.5875)
  line L235 (88.75, 135.5875) -> (101.75, 135.5875)
  arc A232 (88.25, 122.0875) -> (88.75, 121.5875) centre (88.75, 122.0875) ccw
  arc A233 (88.75, 135.5875) -> (88.25, 135.0875) centre (88.75, 135.0875) ccw
  arc A234 (101.75, 121.5875) -> (102.25, 122.0875) centre (101.75, 122.0875) ccw
  arc A235 (102.25, 135.0875) -> (101.75, 135.5875) centre (101.75, 135.0875) ccw
  line L236 (88.25, 141.1375) -> (88.25, 154.1375)
  line L237 (102.25, 141.1375) -> (102.25, 154.1375)
  line L238 (88.75, 140.6375) -> (101.75, 140.6375)
  line L239 (88.75, 154.6375) -> (101.75, 154.6375)
  arc A236 (88.25, 141.1375) -> (88.75, 140.6375) centre (88.75, 141.1375) ccw
  arc A237 (88.75, 154.6375) -> (88.25, 154.1375) centre (88.75, 154.1375) ccw
  arc A238 (101.75, 140.6375) -> (102.25, 141.1375) centre (101.75, 141.1375) ccw
  arc A239 (102.25, 154.1375) -> (101.75, 154.6375) centre (101.75, 154.1375) ccw
  line L240 (88.25, 160.1875) -> (88.25, 173.1875)
  line L241 (102.25, 160.1875) -> (102.25, 173.1875)
  line L242 (88.75, 159.6875) -> (101.75, 159.6875)
  line L243 (88.75, 173.6875) -> (101.75, 173.6875)
  arc A240 (88.25, 160.1875) -> (88.75, 159.6875) centre (88.75, 160.1875) ccw
  arc A241 (88.75, 173.6875) -> (88.25, 173.1875) centre (88.75, 173.1875) ccw
  arc A242 (101.75, 159.6875) -> (102.25, 160.1875) centre (101.75, 160.1875) ccw
  arc A243 (102.25, 173.1875) -> (101.75, 173.6875) centre (101.75, 173.1875) ccw
  line L244 (88.25, 179.2375) -> (88.25, 192.2375)
  line L245 (102.25, 179.2375) -> (102.25, 192.2375)
  line L246 (88.75, 178.7375) -> (101.75, 178.7375)
  line L247 (88.75, 192.7375) -> (101.75, 192.7375)
  arc A244 (88.25, 179.2375) -> (88.75, 178.7375) centre (88.75, 179.2375) ccw
  arc A245 (88.75, 192.7375) -> (88.25, 192.2375) centre (88.75, 192.2375) ccw
  arc A246 (101.75, 178.7375) -> (102.25, 179.2375) centre (101.75, 179.2375) ccw
  arc A247 (102.25, 192.2375) -> (101.75, 192.7375) centre (101.75, 192.2375) ccw
  line L248 (88.25, 198.2875) -> (88.25, 211.2875)
  line L249 (102.25, 198.2875) -> (102.25, 211.2875)
  line L250 (88.75, 197.7875) -> (101.75, 197.7875)
  line L251 (88.75, 211.7875) -> (101.75, 211.7875)
  arc A248 (88.25, 198.2875) -> (88.75, 197.7875) centre (88.75, 198.2875) ccw
  arc A249 (88.75, 211.7875) -> (88.25, 211.2875) centre (88.75, 211.2875) ccw
  arc A250 (101.75, 197.7875) -> (102.25, 198.2875) centre (101.75, 198.2875) ccw
  arc A251 (102.25, 211.2875) -> (101.75, 211.7875) centre (101.75, 211.2875) ccw
  line L252 (88.25, 217.3375) -> (88.25, 230.3375)
  line L253 (102.25, 217.3375) -> (102.25, 230.3375)
  line L254 (88.75, 216.8375) -> (101.75, 216.8375)
  line L255 (88.75, 230.8375) -> (101.75, 230.8375)
  arc A252 (88.25, 217.3375) -> (88.75, 216.8375) centre (88.75, 217.3375) ccw
  arc A253 (88.75, 230.8375) -> (88.25, 230.3375) centre (88.75, 230.3375) ccw
  arc A254 (101.75, 216.8375) -> (102.25, 217.3375) centre (101.75, 217.3375) ccw
  arc A255 (102.25, 230.3375) -> (101.75, 230.8375) centre (101.75, 230.3375) ccw
  line L256 (88.25, 253.0563) -> (88.25, 266.0563)
  line L257 (102.25, 253.0563) -> (102.25, 266.0563)
  line L258 (88.75, 252.5563) -> (101.75, 252.5563)
  line L259 (88.75, 266.5563) -> (101.75, 266.5563)
  arc A256 (88.25, 253.0563) -> (88.75, 252.5563) centre (88.75, 253.0563) ccw
  arc A257 (88.75, 266.5563) -> (88.25, 266.0563) centre (88.75, 266.0563) ccw
  arc A258 (101.75, 252.5563) -> (102.25, 253.0563) centre (101.75, 253.0563) ccw
  arc A259 (102.25, 266.0563) -> (101.75, 266.5563) centre (101.75, 266.0563) ccw
  line L260 (89.25, 244.6183) -> (89.25, 250.6183)
  line L261 (104.25, 244.6183) -> (104.25, 250.6183)
  line L262 (89.75, 244.1183) -> (103.75, 244.1183)
  line L263 (89.75, 251.1183) -> (103.75, 251.1183)
  arc A260 (89.25, 244.6183) -> (89.75, 244.1183) centre (89.75, 244.6183) ccw
  arc A261 (89.75, 251.1183) -> (89.25, 250.6183) centre (89.75, 250.6183) ccw
  arc A262 (103.75, 244.1183) -> (104.25, 244.6183) centre (103.75, 244.6183) ccw
  arc A263 (104.25, 250.6183) -> (103.75, 251.1183) centre (103.75, 250.6183) ccw
  line L264 (89.25, 268.4943) -> (89.25, 274.4943)
  line L265 (104.25, 268.4943) -> (104.25, 274.4943)
  line L266 (89.75, 267.9943) -> (103.75, 267.9943)
  line L267 (89.75, 274.9943) -> (103.75, 274.9943)
  arc A264 (89.25, 268.4943) -> (89.75, 267.9943) centre (89.75, 268.4943) ccw
  arc A265 (89.75, 274.9943) -> (89.25, 274.4943) centre (89.75, 274.4943) ccw
  arc A266 (103.75, 267.9943) -> (104.25, 268.4943) centre (103.75, 268.4943) ccw
  arc A267 (104.25, 274.4943) -> (103.75, 274.9943) centre (103.75, 274.4943) ccw
  line L268 (88.25, 312.5875) -> (88.25, 325.5875)
  line L269 (102.25, 312.5875) -> (102.25, 325.5875)
  line L270 (88.75, 312.0875) -> (101.75, 312.0875)
  line L271 (88.75, 326.0875) -> (101.75, 326.0875)
  arc A268 (88.25, 312.5875) -> (88.75, 312.0875) centre (88.75, 312.5875) ccw
  arc A269 (88.75, 326.0875) -> (88.25, 325.5875) centre (88.75, 325.5875) ccw
  arc A270 (101.75, 312.0875) -> (102.25, 312.5875) centre (101.75, 312.5875) ccw
  arc A271 (102.25, 325.5875) -> (101.75, 326.0875) centre (101.75, 325.5875) ccw
  line L272 (107.3, 5.4062) -> (107.3, 18.4063)
  line L273 (121.3, 5.4063) -> (121.3, 18.4062)
  line L274 (107.8, 4.9063) -> (120.8, 4.9062)
  line L275 (107.8, 18.9063) -> (120.8, 18.9062)
  arc A272 (107.3, 5.4062) -> (107.8, 4.9063) centre (107.8, 5.4063) ccw
  arc A273 (107.8, 18.9062) -> (107.3, 18.4063) centre (107.8, 18.4063) ccw
  arc A274 (120.8, 4.9062) -> (121.3, 5.4063) centre (120.8, 5.4062) ccw
  arc A275 (121.3, 18.4062) -> (120.8, 18.9062) centre (120.8, 18.4062) ccw
  line L276 (107.3, 29.2188) -> (107.3, 42.2188)
  line L277 (121.3, 29.2187) -> (121.3, 42.2188)
  line L278 (107.8, 28.7188) -> (120.8, 28.7188)
  line L279 (107.8, 42.7188) -> (120.8, 42.7188)
  arc A276 (107.3, 29.2188) -> (107.8, 28.7188) centre (107.8, 29.2188) ccw
  arc A277 (107.8, 42.7188) -> (107.3, 42.2187) centre (107.8, 42.2188) ccw
  arc A278 (120.8, 28.7188) -> (121.3, 29.2188) centre (120.8, 29.2187) ccw
  arc A279 (121.3, 42.2188) -> (120.8, 42.7188) centre (120.8, 42.2188) ccw
  line L280 (107.3, 53.0313) -> (107.3, 66.0313)
  line L281 (121.3, 53.0313) -> (121.3, 66.0312)
  line L282 (107.8, 52.5312) -> (120.8, 52.5313)
  line L283 (107.8, 66.5313) -> (120.8, 66.5312)
  arc A280 (107.3, 53.0313) -> (107.8, 52.5312) centre (107.8, 53.0312) ccw
  arc A281 (107.8, 66.5313) -> (107.3, 66.0313) centre (107.8, 66.0312) ccw
  arc A282 (120.8, 52.5313) -> (121.3, 53.0313) centre (120.8, 53.0313) ccw
  arc A283 (121.3, 66.0312) -> (120.8, 66.5312) centre (120.8, 66.0313) ccw
  line L284 (107.3, 124.4688) -> (107.3, 137.4688)
  line L285 (121.3, 124.4688) -> (121.3, 137.4688)
  line L286 (107.8, 123.9688) -> (120.8, 123.9688)
  line L287 (107.8, 137.9688) -> (120.8, 137.9688)
  arc A284 (107.3, 124.4688) -> (107.8, 123.9688) centre (107.8, 124.4688) ccw
  arc A285 (107.8, 137.9688) -> (107.3, 137.4688) centre (107.8, 137.4688) ccw
  arc A286 (120.8, 123.9688) -> (121.3, 124.4688) centre (120.8, 124.4688) ccw
  arc A287 (121.3, 137.4688) -> (120.8, 137.9688) centre (120.8, 137.4688) ccw
  line L288 (108.3, 77.9688) -> (108.3, 83.9688)
  line L289 (123.3, 77.9688) -> (123.3, 83.9688)
  line L290 (108.8, 77.4688) -> (122.8, 77.4688)
  line L291 (108.8, 84.4688) -> (122.8, 84.4688)
  arc A288 (108.3, 77.9688) -> (108.8, 77.4688) centre (108.8, 77.9688) ccw
  arc A289 (108.8, 84.4688) -> (108.3, 83.9688) centre (108.8, 83.9688) ccw
  arc A290 (122.8, 77.4688) -> (123.3, 77.9688) centre (122.8, 77.9688) ccw
  arc A291 (123.3, 83.9688) -> (122.8, 84.4688) centre (122.8, 83.9688) ccw
  line L292 (108.3, 177.9688) -> (108.3, 183.9688)
  line L293 (123.3, 177.9688) -> (123.3, 183.9688)
  line L294 (108.8, 177.4688) -> (122.8, 177.4688)
  line L295 (108.8, 184.4688) -> (122.8, 184.4688)
  arc A292 (108.3, 177.9688) -> (108.8, 177.4688) centre (108.8, 177.9688) ccw
  arc A293 (108.8, 184.4688) -> (108.3, 183.9688) centre (108.8, 183.9688) ccw
  arc A294 (122.8, 177.4688) -> (123.3, 177.9688) centre (122.8, 177.9688) ccw
  arc A295 (123.3, 183.9688) -> (122.8, 184.4688) centre (122.8, 183.9688) ccw
  line L296 (107.3, 195.9063) -> (107.3, 208.9063)
  line L297 (121.3, 195.9063) -> (121.3, 208.9063)
  line L298 (107.8, 195.4063) -> (120.8, 195.4063)
  line L299 (107.8, 209.4063) -> (120.8, 209.4063)
  arc A296 (107.3, 195.9063) -> (107.8, 195.4063) centre (107.8, 195.9063) ccw
  arc A297 (107.8, 209.4063) -> (107.3, 208.9063) centre (107.8, 208.9063) ccw
  arc A298 (120.8, 195.4063) -> (121.3, 195.9063) centre (120.8, 195.9063) ccw
  arc A299 (121.3, 208.9063) -> (120.8, 209.4063) centre (120.8, 208.9063) ccw
  line L300 (107.3, 219.7188) -> (107.3, 232.7188)
  line L301 (121.3, 219.7188) -> (121.3, 232.7188)
  line L302 (107.8, 219.2188) -> (120.8, 219.2188)
  line L303 (107.8, 233.2188) -> (120.8, 233.2188)
  arc A300 (107.3, 219.7188) -> (107.8, 219.2188) centre (107.8, 219.7188) ccw
  arc A301 (107.8, 233.2188) -> (107.3, 232.7188) centre (107.8, 232.7188) ccw
  arc A302 (120.8, 219.2188) -> (121.3, 219.7188) centre (120.8, 219.7188) ccw
  arc A303 (121.3, 232.7188) -> (120.8, 233.2188) centre (120.8, 232.7188) ccw
  line L304 (107.3, 243.5313) -> (107.3, 256.5313)
  line L305 (121.3, 243.5313) -> (121.3, 256.5313)
  line L306 (107.8, 243.0313) -> (120.8, 243.0313)
  line L307 (107.8, 257.0313) -> (120.8, 257.0313)
  arc A304 (107.3, 243.5313) -> (107.8, 243.0313) centre (107.8, 243.5313) ccw
  arc A305 (107.8, 257.0313) -> (107.3, 256.5313) centre (107.8, 256.5313) ccw
  arc A306 (120.8, 243.0313) -> (121.3, 243.5313) centre (120.8, 243.5313) ccw
  arc A307 (121.3, 256.5313) -> (120.8, 257.0313) centre (120.8, 256.5313) ccw
  line L308 (107.3, 267.3438) -> (107.3, 280.3438)
  line L309 (121.3, 267.3438) -> (121.3, 280.3438)
  line L310 (107.8, 266.8438) -> (120.8, 266.8438)
  line L311 (107.8, 280.8438) -> (120.8, 280.8438)
  arc A308 (107.3, 267.3438) -> (107.8, 266.8438) centre (107.8, 267.3438) ccw
  arc A309 (107.8, 280.8438) -> (107.3, 280.3438) centre (107.8, 280.3438) ccw
  arc A310 (120.8, 266.8438) -> (121.3, 267.3438) centre (120.8, 267.3438) ccw
  arc A311 (121.3, 280.3438) -> (120.8, 280.8438) centre (120.8, 280.3438) ccw
  line L312 (107.3, 293.5375) -> (107.3, 306.5375)
  line L313 (121.3, 293.5375) -> (121.3, 306.5375)
  line L314 (107.8, 293.0375) -> (120.8, 293.0375)
  line L315 (107.8, 307.0375) -> (120.8, 307.0375)
  arc A312 (107.3, 293.5375) -> (107.8, 293.0375) centre (107.8, 293.5375) ccw
  arc A313 (107.8, 307.0375) -> (107.3, 306.5375) centre (107.8, 306.5375) ccw
  arc A314 (120.8, 293.0375) -> (121.3, 293.5375) centre (120.8, 293.5375) ccw
  arc A315 (121.3, 306.5375) -> (120.8, 307.0375) centre (120.8, 306.5375) ccw
  line L316 (107.3, 312.5875) -> (107.3, 325.5875)
  line L317 (121.3, 312.5875) -> (121.3, 325.5875)
  line L318 (107.8, 312.0875) -> (120.8, 312.0875)
  line L319 (107.8, 326.0875) -> (120.8, 326.0875)
  arc A316 (107.3, 312.5875) -> (107.8, 312.0875) centre (107.8, 312.5875) ccw
  arc A317 (107.8, 326.0875) -> (107.3, 325.5875) centre (107.8, 325.5875) ccw
  arc A318 (120.8, 312.0875) -> (121.3, 312.5875) centre (120.8, 312.5875) ccw
  arc A319 (121.3, 325.5875) -> (120.8, 326.0875) centre (120.8, 325.5875) ccw
  line L320 (107.3, 331.6375) -> (107.3, 344.6375)
  line L321 (121.3, 331.6375) -> (121.3, 344.6375)
  line L322 (107.8, 331.1375) -> (120.8, 331.1375)
  line L323 (107.8, 345.1375) -> (120.8, 345.1375)
  arc A320 (107.3, 331.6375) -> (107.8, 331.1375) centre (107.8, 331.6375) ccw
  arc A321 (107.8, 345.1375) -> (107.3, 344.6375) centre (107.8, 344.6375) ccw
  arc A322 (120.8, 331.1375) -> (121.3, 331.6375) centre (120.8, 331.6375) ccw
  arc A323 (121.3, 344.6375) -> (120.8, 345.1375) centre (120.8, 344.6375) ccw
  point P0 (73.563, 167.981)
sketch "Block2" plane through (0, 0, 0) normal (0, 0, 1) x (1, 0, 0)
  line L0 (2.525, 3.025) -> (2.525, 16.025)
  line L1 (16.525, 3.025) -> (16.525, 16.025)
  line L2 (3.025, 2.525) -> (16.025, 2.525)
  line L3 (3.025, 16.525) -> (16.025, 16.525)
  arc A0 (2.525, 3.025) -> (3.025, 2.525) centre (3.025, 3.025) ccw
  arc A1 (3.025, 16.525) -> (2.525, 16.025) centre (3.025, 16.025) ccw
  arc A2 (16.025, 2.525) -> (16.525, 3.025) centre (16.025, 3.025) ccw
  arc A3 (16.525, 16.025) -> (16.025, 16.525) centre (16.025, 16.025) ccw
  line L4 (2.525, 41.125) -> (2.525, 54.125)
  line L5 (16.525, 41.125) -> (16.525, 54.125)
  line L6 (3.025, 40.625) -> (16.025, 40.625)
  line L7 (3.025, 54.625) -> (16.025, 54.625)
  arc A4 (2.525, 41.125) -> (3.025, 40.625) centre (3.025, 41.125) ccw
  arc A5 (3.025, 54.625) -> (2.525, 54.125) centre (3.025, 54.125) ccw
  arc A6 (16.025, 40.625) -> (16.525, 41.125) centre (16.025, 41.125) ccw
  arc A7 (16.525, 54.125) -> (16.025, 54.625) centre (16.025, 54.125) ccw
  line L8 (2.525, 60.175) -> (2.525, 73.175)
  line L9 (16.525, 60.175) -> (16.525, 73.175)
  line L10 (3.025, 59.675) -> (16.025, 59.675)
  line L11 (3.025, 73.675) -> (16.025, 73.675)
  arc A8 (2.525, 60.175) -> (3.025, 59.675) centre (3.025, 60.175) ccw
  arc A9 (3.025, 73.675) -> (2.525, 73.175) centre (3.025, 73.175) ccw
  arc A10 (16.025, 59.675) -> (16.525, 60.175) centre (16.025, 60.175) ccw
  arc A11 (16.525, 73.175) -> (16.025, 73.675) centre (16.025, 73.175) ccw
  line L12 (2.525, 79.225) -> (2.525, 92.225)
  line L13 (16.525, 79.225) -> (16.525, 92.225)
  line L14 (3.025, 78.725) -> (16.025, 78.725)
  line L15 (3.025, 92.725) -> (16.025, 92.725)
  arc A12 (2.525, 79.225) -> (3.025, 78.725) centre (3.025, 79.225) ccw
  arc A13 (3.025, 92.725) -> (2.525, 92.225) centre (3.025, 92.225) ccw
  arc A14 (16.025, 78.725) -> (16.525, 79.225) centre (16.025, 79.225) ccw
  arc A15 (16.525, 92.225) -> (16.025, 92.725) centre (16.025, 92.225) ccw
  line L16 (2.525, 98.275) -> (2.525, 111.275)
  line L17 (16.525, 98.275) -> (16.525, 111.275)
  line L18 (3.025, 97.775) -> (16.025, 97.775)
  line L19 (3.025, 111.775) -> (16.025, 111.775)
  arc A16 (2.525, 98.275) -> (3.025, 97.775) centre (3.025, 98.275) ccw
  arc A17 (3.025, 111.775) -> (2.525, 111.275) centre (3.025, 111.275) ccw
  arc A18 (16.025, 97.775) -> (16.525, 98.275) centre (16.025, 98.275) ccw
  arc A19 (16.525, 111.275) -> (16.025, 111.775) centre (16.025, 111.275) ccw
  line L20 (2.525, 126.85) -> (2.525, 139.85)
  line L21 (16.525, 126.85) -> (16.525, 139.85)
  line L22 (3.025, 126.35) -> (16.025, 126.35)
  line L23 (3.025, 140.35) -> (16.025, 140.35)
  arc A20 (2.525, 126.85) -> (3.025, 126.35) centre (3.025, 126.85) ccw
  arc A21 (3.025, 140.35) -> (2.525, 139.85) centre (3.025, 139.85) ccw
  arc A22 (16.025, 126.35) -> (16.525, 126.85) centre (16.025, 126.85) ccw
  arc A23 (16.525, 139.85) -> (16.025, 140.35) centre (16.025, 139.85) ccw
  line L24 (2.525, 145.9) -> (2.525, 158.9)
  line L25 (16.525, 145.9) -> (16.525, 158.9)
  line L26 (3.025, 145.4) -> (16.025, 145.4)
  line L27 (3.025, 159.4) -> (16.025, 159.4)
  arc A24 (2.525, 145.9) -> (3.025, 145.4) centre (3.025, 145.9) ccw
  arc A25 (3.025, 159.4) -> (2.525, 158.9) centre (3.025, 158.9) ccw
  arc A26 (16.025, 145.4) -> (16.525, 145.9) centre (16.025, 145.9) ccw
  arc A27 (16.525, 158.9) -> (16.025, 159.4) centre (16.025, 158.9) ccw
  line L28 (2.525, 164.95) -> (2.525, 177.95)
  line L29 (16.525, 164.95) -> (16.525, 177.95)
  line L30 (3.025, 164.45) -> (16.025, 164.45)
  line L31 (3.025, 178.45) -> (16.025, 178.45)
  arc A28 (2.525, 164.95) -> (3.025, 164.45) centre (3.025, 164.95) ccw
  arc A29 (3.025, 178.45) -> (2.525, 177.95) centre (3.025, 177.95) ccw
  arc A30 (16.025, 164.45) -> (16.525, 164.95) centre (16.025, 164.95) ccw
  arc A31 (16.525, 177.95) -> (16.025, 178.45) centre (16.025, 177.95) ccw
  line L32 (2.525, 184) -> (2.525, 197)
  line L33 (16.525, 184) -> (16.525, 197)
  line L34 (3.025, 183.5) -> (16.025, 183.5)
  line L35 (3.025, 197.5) -> (16.025, 197.5)
  arc A32 (2.525, 184) -> (3.025, 183.5) centre (3.025, 184) ccw
  arc A33 (3.025, 197.5) -> (2.525, 197) centre (3.025, 197) ccw
  arc A34 (16.025, 183.5) -> (16.525, 184) centre (16.025, 184) ccw
  arc A35 (16.525, 197) -> (16.025, 197.5) centre (16.025, 197) ccw
  line L36 (2.525, 212.575) -> (2.525, 225.575)
  line L37 (16.525, 212.575) -> (16.525, 225.575)
  line L38 (3.025, 212.075) -> (16.025, 212.075)
  line L39 (3.025, 226.075) -> (16.025, 226.075)
  arc A36 (2.525, 212.575) -> (3.025, 212.075) centre (3.025, 212.575) ccw
  arc A37 (3.025, 226.075) -> (2.525, 225.575) centre (3.025, 225.575) ccw
  arc A38 (16.025, 212.075) -> (16.525, 212.575) centre (16.025, 212.575) ccw
  arc A39 (16.525, 225.575) -> (16.025, 226.075) centre (16.025, 225.575) ccw
  line L40 (2.525, 231.625) -> (2.525, 244.625)
  line L41 (16.525, 231.625) -> (16.525, 244.625)
  line L42 (3.025, 231.125) -> (16.025, 231.125)
  line L43 (3.025, 245.125) -> (16.025, 245.125)
  arc A40 (2.525, 231.625) -> (3.025, 231.125) centre (3.025, 231.625) ccw
  arc A41 (3.025, 245.125) -> (2.525, 244.625) centre (3.025, 244.625) ccw
  arc A42 (16.025, 231.125) -> (16.525, 231.625) centre (16.025, 231.625) ccw
  arc A43 (16.525, 244.625) -> (16.025, 245.125) centre (16.025, 244.625) ccw
  line L44 (2.525, 250.675) -> (2.525, 263.675)
  line L45 (16.525, 250.675) -> (16.525, 263.675)
  line L46 (3.025, 250.175) -> (16.025, 250.175)
  line L47 (3.025, 264.175) -> (16.025, 264.175)
  arc A44 (2.525, 250.675) -> (3.025, 250.175) centre (3.025, 250.675) ccw
  arc A45 (3.025, 264.175) -> (2.525, 263.675) centre (3.025, 263.675) ccw
  arc A46 (16.025, 250.175) -> (16.525, 250.675) centre (16.025, 250.675) ccw
  arc A47 (16.525, 263.675) -> (16.025, 264.175) centre (16.025, 263.675) ccw
  line L48 (2.525, 269.725) -> (2.525, 282.725)
  line L49 (16.525, 269.725) -> (16.525, 282.725)
  line L50 (3.025, 269.225) -> (16.025, 269.225)
  line L51 (3.025, 283.225) -> (16.025, 283.225)
  arc A48 (2.525, 269.725) -> (3.025, 269.225) centre (3.025, 269.725) ccw
  arc A49 (3.025, 283.225) -> (2.525, 282.725) centre (3.025, 282.725) ccw
  arc A50 (16.025, 269.225) -> (16.525, 269.725) centre (16.025, 269.725) ccw
  arc A51 (16.525, 282.725) -> (16.025, 283.225) centre (16.025, 282.725) ccw
  point P0 (9.525, 150.2019)